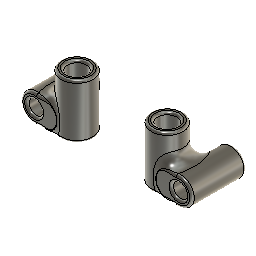
2-Attaches_base_V_arriere (Autodesk Fusion 360 design; units mm, degrees)
Autodesk Fusion 360 part; units mm, degrees
sketch "Sketch1" plane through (0, 0, 0) normal (0, 0, 1) x (1, 0, 0)
  circle A0 centre (0, 0) radius 2.1
  circle A1 centre (0, 0) radius 3.5
  dimension "d1" = 4.2
  dimension "d2" = 7
  measures "d1" diameter of A0
  measures "d2" diameter of A1
extrude "Extrude1" add sketch "Sketch1" along normal blind 12 makes body 1
ref_plane "WorkPlane1" through (3.25, 0, 0) normal (1, 0, 0) x (0, 1, 0)
sketch "Sketch2" plane through (3.25, 0, 0) normal (1, 0, 0) x (0, 1, 0)
ref_plane "WorkPlane2" through (0, -3.25, 0) normal (0, 1, 0) x (0, 0, 1)
sketch "Sketch3" plane through (0, -3.25, 0) normal (0, 1, 0) x (1, 0, 0)
ref_plane "WorkPlane3" through (0, -3.5, 0) normal (0, 1, 0) x (0, 0, 1)
sketch "Sketch4" plane through (0, -3.5, 0) normal (0, 1, 0) x (1, 0, 0)
  circle A0 centre (6, -3) radius 3
  circle A1 centre (6, -3) radius 1.6
  dimension "d10" = 3.2
  dimension "d11" = 6
  measures "d10" diameter of A1
  measures "d11" diameter of A0
extrude "Extrude2" add sketch "Sketch4" along normal blind 12 bodies 1
fillet "Fillet1" radius 2.4 1 edges at (3.5, 0, 4.6583) on bodies 1
fillet "Fillet2" radius 0.5 1 edges at (-1.9579, 0.7594, 12) on bodies 1
fillet "Fillet3" radius 0.5 1 edges at (-3.2631, -1.2657, 12) on bodies 1
fillet "Fillet4" radius 0.5 3 edges at (4.7745, -2.4574, 0) (4.0726, 2.9256, 0) (-3.5, 0, 0) on bodies 1
fillet "Fillet5" radius 0.5 1 edges at (3.203, 8.5, 4.0848) on bodies 1
fillet "Fillet6" radius 0.5 1 edges at (4.5083, 8.5, 2.4214) on bodies 1
fillet "Fillet7" radius 0.5 1 edges at (4.5083, -3.5, 2.4214) on bodies 1
fillet "Fillet8" radius 0.5 2 edges at (1.0142, -3.5, 3.433) (9, -3.5, 3) on bodies 1
fillet "Fillet9" radius 0.5 1 edges at (-1.9579, 0.7594, 0) on bodies 1
ref_plane "WorkPlane4" through (-10, 0, 0) normal (1, 0, 0) x (0, 1, 0)
mirror "Mirror1" about plane through (-10, 0, 0) normal (1, 0, 0) of bodies 1 makes body 2
